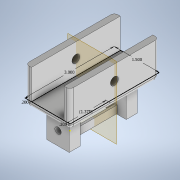
# Autodesk Inventor part: Capillary Holder with O-ring system_rev3_dblOring
Saved by Autodesk Inventor 2020 (Build 240168000, 168)
## iProperties
Created: 2022-02-15
Part Number: Capillary Holder with O-ring system_rev3_dblOring
Material: Generic
Document SubType Name: Modeling
Designer: Beaucage
Density: 1 g/cm^3
Appearance: Default
Author: Beaucage
Autodesk Inventor part; units mm, degrees
ref_plane "YZ Plane" through (0, 0, 0) normal (1, 0, 0) x (0, 1, 0)
ref_plane "XZ Plane" through (0, 0, 0) normal (0, 1, 0) x (-1, 0, 0)
sketch "Sketch1" plane through (0, 0, 0) normal (0, 1, 0) x (-1, 0, 0)
  line L0 (0, 0) -> (38.1, 0)
  line L1 (38.1, 0) -> (38.1, -76.2)
  line L2 (38.1, -76.2) -> (0, -76.2)
  line L3 (0, -76.2) -> (0, 0)
  line L4 (38.1, -76.2) -> (33.02, -76.2)
  line L5 (33.02, -76.2) -> (33.02, 0)
  line L6 (33.02, 0) -> (38.1, 0)
  line L7 (38.1, 0) -> (38.1, -76.2)
  line L8 (0, -76.2) -> (5.08, -76.2)
  line L9 (5.08, -76.2) -> (5.08, 0)
  line L10 (5.08, 0) -> (0, 0)
  line L11 (0, 0) -> (0, -76.2)
  dimension "d0" = 38.1
  dimension "d1" = 76.2
  dimension "d2" = 5.08
  dimension "d3" = 5.08
  constraints: 24 end point, 6 parallel, 3 horizontal, 3 perpendicular, 2 point on line
  measures "d0" distance of L1.end L2.end
  measures "d1" distance of L0.end L1.end
  measures "d2" distance of L5.end L6.end
  measures "d3" distance of L10.end L9.end
extrude "Extrusion1" add sketch "Sketch1" along normal blind 25.4 contours L0 L9 L2 L3 | L0 L1 L2 L5
extrude "Extrusion2" add sketch "Sketch1" against normal blind 5.08
sketch "Sketch2" plane through (0, 25.4, 0) normal (1, 0, 0) x (0, 0, -1)
  line L0 (76.2, 0) -> (0, 0) projected
  line L1 (38.1, 0) -> (38.1, -12.7)
  point P0 (0, -25.4)
  dimension "d8" = 12.7
  constraints: 2 end point, 1 midpoint, 1 vertical
  measures "d8" distance of L1.start L1.end
hole "Hole1" at (0, 12.7, -38.1) direction (-1, 0, 0) diameter 6.7564 end through all clearance for "Socket Head Cap Screw" size "1/4" standard "Ansi Unified Screw Threads"
sketch "Sketch3" plane through (0, -5.08, 0) normal (0, -1, 0) x (1, 0, 0)
  line L0 (0, -76.2) -> (-5.08, -76.2) projected
  line L1 (0, -76.2) -> (0, -63.5)
  line L2 (0, 0) -> (0, -76.2) projected
  line L3 (0, -63.5) -> (0, -38.1)
  line L4 (0, -63.5) -> (-19.05, -63.5)
  line L5 (0, -38.1) -> (-19.05, -38.1)
  line L6 (-38.1, -76.2) -> (-38.1, 0) projected
  line L7 (0, -65.0875) -> (-38.1, -65.0875)
  line L8 (-38.1, -65.0875) -> (-38.1, -61.9125)
  line L9 (-38.1, -61.9125) -> (0, -61.9125)
  line L10 (0, -61.9125) -> (0, -65.0875)
  line L11 (0, -65.0875) -> (-38.1, -61.9125) construction
  line L12 (-38.1, -65.0875) -> (0, -61.9125) construction
  line L13 (0, -36.5125) -> (-38.1, -36.5125)
  line L14 (-38.1, -36.5125) -> (-38.1, -39.6875)
  line L15 (-38.1, -39.6875) -> (0, -39.6875)
  line L16 (0, -39.6875) -> (0, -36.5125)
  line L17 (0, -36.5125) -> (-38.1, -39.6875) construction
  line L18 (-38.1, -36.5125) -> (0, -39.6875) construction
  line L19 (-38.1, 0) -> (-38.1, -76.2) projected
  line L20 (-38.1, 0) -> (0, 0)
  line L21 (0, 0) -> (0, -3.175)
  line L22 (0, -3.175) -> (-38.1, -3.175)
  line L23 (-38.1, -3.175) -> (-38.1, 0)
  line L24 (0, -76.2) -> (-38.1, -76.2)
  line L25 (-38.1, -76.2) -> (-38.1, -73.025)
  line L26 (-38.1, -73.025) -> (0, -73.025)
  line L27 (0, -73.025) -> (0, -76.2)
  line L28 (0, -3.175) -> (0, -15.875)
  line L29 (-38.1, -73.025) -> (-38.1, -60.325)
  line L30 (-38.1, -73.025) -> (-25.4, -73.025) construction
  line L31 (0, -15.875) -> (-38.1, -15.875)
  line L32 (-38.1, -15.875) -> (-38.1, -18.415)
  line L33 (-38.1, -18.415) -> (0, -18.415)
  line L34 (0, -18.415) -> (0, -15.875)
  line L35 (-38.1, -60.325) -> (0.7144, -60.325)
  line L36 (0.7144, -60.325) -> (0.7144, -57.785)
  line L37 (0.7144, -57.785) -> (-38.1, -57.785)
  line L38 (-38.1, -57.785) -> (-38.1, -60.325)
  line L39 (-33.02, 0) -> (-5.08, 0) projected
  line L40 (-38.1, -3.175) -> (-25.4, -3.175)
  line L41 (-25.4, -3.175) -> (-25.4, 0)
  line L42 (-25.4, 0) -> (-38.1, 0)
  line L43 (-38.1, 0) -> (-38.1, -3.175)
  line L44 (0, -3.175) -> (-12.7, -3.175)
  line L45 (-12.7, -3.175) -> (-12.7, 0)
  line L46 (-12.7, 0) -> (0, 0)
  line L47 (0, 0) -> (0, -3.175)
  line L48 (-38.1, -76.2) -> (-25.4, -76.2)
  line L49 (-25.4, -76.2) -> (-25.4, -73.025)
  line L50 (-25.4, -73.025) -> (-38.1, -73.025)
  line L51 (-38.1, -73.025) -> (-38.1, -76.2)
  line L52 (0, -76.2) -> (-12.7, -76.2)
  line L53 (-12.7, -76.2) -> (-12.7, -73.025)
  line L54 (-12.7, -73.025) -> (0, -73.025)
  line L55 (0, -73.025) -> (0, -76.2)
  line L56 (0, -15.875) -> (-9.525, -15.875)
  line L57 (-9.525, -15.875) -> (-9.525, -18.415)
  line L58 (-9.525, -18.415) -> (0, -18.415)
  line L59 (0, -18.415) -> (0, -15.875)
  line L60 (0, -57.785) -> (-9.525, -57.785)
  line L61 (-9.525, -57.785) -> (-9.525, -60.325)
  line L62 (-9.525, -60.325) -> (0, -60.325)
  line L63 (0, -60.325) -> (0, -57.785)
  line L64 (-38.1, -18.415) -> (-28.575, -18.415)
  line L65 (-28.575, -18.415) -> (-28.575, -15.875)
  line L66 (-28.575, -15.875) -> (-38.1, -15.875)
  line L67 (-38.1, -15.875) -> (-38.1, -18.415)
  line L68 (-28.575, -57.785) -> (-38.1, -57.785)
  line L69 (-38.1, -57.785) -> (-38.1, -60.325)
  line L70 (-38.1, -60.325) -> (-28.575, -60.325)
  line L71 (-28.575, -60.325) -> (-28.575, -57.785)
  line L72 (-9.525, -18.415) -> (-28.575, -18.415)
  line L73 (-28.575, -18.415) -> (-28.575, -8.89)
  line L74 (-28.575, -8.89) -> (-9.525, -8.89)
  line L75 (-9.525, -8.89) -> (-9.525, -18.415)
  line L76 (-28.575, -57.785) -> (-9.525, -57.785)
  line L77 (-9.525, -57.785) -> (-9.525, -67.31)
  line L78 (-9.525, -67.31) -> (-28.575, -67.31)
  line L79 (-28.575, -67.31) -> (-28.575, -57.785)
  point P0 (0, -39.6875)
  point P1 (0, -36.5125)
  point P2 (-38.1, -36.5125)
  point P3 (0, -61.9125)
  point P4 (-38.1, -65.0875)
  point P5 (0, -65.0875)
  point P6 (0, -73.025)
  point P7 (-38.1, -18.415)
  point P8 (0, -18.415)
  point P9 (-38.1, -15.875)
  point P10 (0, -57.785)
  point P11 (0, -60.325)
  dimension "d16" = 12.7
  dimension "d17" = 25.4
  dimension "d18" = 19.05
  dimension "d19" = 3.175
  dimension "d20" = 3.175
  dimension "d32" = 3.175
  dimension "d33" = 3.175
  dimension "d34" = 12.7
  dimension "d35" = 12.7
  dimension "d36" = 90
  dimension "d37" = 2.54
  dimension "d38" = 2.54
  dimension "d46" = 12.7
  dimension "d47" = 12.7
  dimension "d48" = 12.7
  dimension "d49" = 9.525
  dimension "d50" = 9.525
  dimension "d51" = 9.525
  constraints: 150 end point, 32 parallel, 19 horizontal, 17 perpendicular, 17 point on line, 5 midpoint, 1 collinear, 3 other
  measures "d16" distance of L0.start L1.end
  measures "d17" distance of L1.end L3.end
  measures "d18" distance of L1.end L4.end
  measures "d19" distance of L7.end L8.end
  measures "d20" distance of L14.end L13.end
  measures "d32" distance of L20.end L21.end
  measures "d33" distance of L24.end L25.end
  measures "d34" distance of L21.end L28.end
  measures "d35" distance of L25.end L29.end
  measures "d36" angle of L30 L29
  measures "d37" distance of L32.end L31.end
  measures "d38" distance of L36.end L35.end
  measures "d46" distance of L42.end L41.end
  measures "d47" distance of L45.end L46.end
  measures "d48" distance of L50.end L30.end
  measures "d49" distance of L66.end L65.end
  measures "d50" distance of L72.end L73.end
  measures "d51" distance of L76.end L77.end
extrude "Extrusion3" add sketch "Sketch3" along normal blind 25.4 contours L77 L78 L79 L7 | L7 L79 L9 L77 | L9 L79 L35 L77 | L35 L71 L37 L61 | L33 L65 L31 L57 | L31 L73 L74 L75
sketch "Sketch4" plane through (-38.1, -5.08, 0) normal (0, 0, 1) x (1, 0, 0)
  line L0 (38.1, -25.4) -> (19.05, -25.4)
  line L1 (19.05, -25.4) -> (19.05, -13.97)
  point P0 (38.1, 5.08)
  dimension "d23" = 11.43
  constraints: 4 end point, 1 vertical
  measures "d23" distance of L0.end L1.end
hole "Hole2" at (-19.05, -19.05, 0) direction (0, 0, -1) diameter 2 end through all
fillet "Fillet1" radius 3.175 8 edges at (-38.1, 10.16, 0) (-19.05, -5.08, 0) (0, 10.16, 0) (-19.05, -5.08, -76.2) (0, 10.16, -76.2) (-38.1, 10.16, -76.2) (0, -5.08, -38.1) (-38.1, -5.08, -38.1)
sketch "Sketch5" plane through (-38.1, -30.48, -57.785) normal (0, 0, 1) x (1, 0, 0)
  line L0 (28.575, 0) -> (9.525, 0) projected
  line L1 (19.05, 0) -> (19.05, 3.175)
  line L2 (19.05, 0.7419) -> (20.955, 0.7419)
  line L3 (20.955, 0.7419) -> (20.955, 7.0919)
  line L4 (20.955, 7.0919) -> (19.05, 7.0919)
  line L5 (19.05, 7.0919) -> (19.05, 0.7419)
  point P0 (38.1, 30.48)
  point P1 (38.8144, 0)
  point P2 (0, 0)
  point P3 (38.1, 0)
  dimension "d39" = 3.175
  dimension "d40" = 1.905
  dimension "d41" = 6.35
  constraints: 10 end point, 2 parallel, 1 horizontal, 1 midpoint, 1 perpendicular, 1 point on line, 1 vertical
  measures "d39" distance of L1.start L1.end
  measures "d40" distance of L4.end L3.end
  measures "d41" distance of L3.end L2.end
extrude "Extrusion4" add sketch "Sketch5" along normal blind 40.64
sketch "Sketch6" plane through (-19.05, -29.7381, -57.785) normal (-1, 0, 0) x (0, 0, 1)
  line L0 (38.4322, 1.5042) -> (1.8474, 1.5042) construction
  line L1 (1.8474, 1.5042) -> (1.8474, 6.5412) construction
  line L2 (1.8474, 6.5412) -> (38.4322, 6.5412) construction
  line L3 (38.4322, 6.5412) -> (38.4322, 1.5042) construction
  spline S0 degree 2 poles (36.9329, 4.7424) (37.2293, 4.7424) (37.7307, 4.5423) (37.9135, 4.3422) knots 0 0 0 1 2 2 2
  spline S1 degree 2 poles (37.9135, 4.3422) (38.0963, 4.1446) (38.2963, 3.5518) (38.2963, 3.1665) knots 0 0 0 1 2 2 2
  spline S2 degree 2 poles (38.2963, 3.1665) (38.2963, 2.7836) (38.1012, 2.2155) (37.916, 2.0056) knots 0 0 0 1 2 2 2
  spline S3 degree 2 poles (37.916, 2.0056) (37.7332, 1.8006) (37.2342, 1.5857) (36.9255, 1.5857) knots 0 0 0 1 2 2 2
  spline S4 degree 2 poles (36.9255, 1.5857) (36.7723, 1.5857) (36.5031, 1.6302) (36.3895, 1.6647) knots 0 0 0 1 2 2 2
  spline S5 degree 2 poles (36.3895, 1.6647) (36.2907, 1.6968) (36.0857, 1.7882) (35.9844, 1.8426) knots 0 0 0 1 2 2 2
  line L4 (35.9844, 1.8426) -> (35.9844, 2.3316)
  line L5 (35.9844, 2.3316) -> (36.0165, 2.3316)
  spline S6 degree 2 poles (36.0165, 2.3316) (36.0709, 2.2822) (36.2388, 2.1439) (36.3598, 2.0772) knots 0 0 0 1 2 2 2
  spline S7 degree 2 poles (36.3598, 2.0772) (36.4759, 2.013) (36.7501, 1.9315) (36.9279, 1.9315) knots 0 0 0 1 2 2 2
  spline S8 degree 2 poles (36.9279, 1.9315) (37.1231, 1.9315) (37.4714, 2.092) (37.6023, 2.2452) knots 0 0 0 1 2 2 2
  spline S9 degree 2 poles (37.6023, 2.2452) (37.7307, 2.4008) (37.874, 2.8726) (37.874, 3.1665) knots 0 0 0 1 2 2 2
  spline S10 degree 2 poles (37.874, 3.1665) (37.874, 3.4802) (37.7233, 3.9322) (37.5924, 4.0878) knots 0 0 0 1 2 2 2
  spline S11 degree 2 poles (37.5924, 4.0878) (37.4639, 4.2385) (37.1206, 4.3916) (36.9279, 4.3916) knots 0 0 0 1 2 2 2
  spline S12 degree 2 poles (36.9279, 4.3916) (36.7526, 4.3916) (36.4537, 4.3052) (36.3376, 4.241) knots 0 0 0 1 2 2 2
  spline S13 degree 2 poles (36.3376, 4.241) (36.2265, 4.1767) (36.061, 4.0434) (36.014, 3.9964) knots 0 0 0 1 2 2 2
  line L6 (36.014, 3.9964) -> (35.9844, 3.9964)
  line L7 (35.9844, 3.9964) -> (35.9844, 4.4805)
  spline S14 degree 2 poles (35.9844, 4.4805) (36.0857, 4.5275) (36.2635, 4.6139) (36.3895, 4.6535) knots 0 0 0 1 2 2 2
  spline S15 degree 2 poles (36.3895, 4.6535) (36.5229, 4.6979) (36.7501, 4.7424) (36.9329, 4.7424) knots 0 0 0 1 2 2 2
  spline S16 degree 2 poles (34.3616, 4.446) (34.4085, 4.4805) (34.5666, 4.6041) (34.6407, 4.6411) knots 0 0 0 1 2 2 2
  spline S17 degree 2 poles (34.6407, 4.6411) (34.742, 4.6954) (34.9322, 4.7523) (35.1051, 4.7523) knots 0 0 0 1 2 2 2
  spline S18 degree 2 poles (35.1051, 4.7523) (35.2459, 4.7523) (35.5003, 4.646) (35.5966, 4.5497) knots 0 0 0 1 2 2 2
  spline S19 degree 2 poles (35.5966, 4.5497) (35.688, 4.4558) (35.7991, 4.1792) (35.7991, 4.0261) knots 0 0 0 1 2 2 2
  spline S20 degree 2 poles (35.7991, 4.0261) (35.7991, 3.7889) (35.5991, 3.453) (35.3817, 3.3567) knots 0 0 0 1 2 2 2
  spline S21 degree 2 poles (35.3817, 3.3567) (35.1891, 3.2678) (34.6654, 3.2011) (34.3616, 3.1838) knots 0 0 0 1 2 2 2
  line L8 (34.3616, 3.1838) -> (34.3616, 3.1097)
  spline S22 degree 2 poles (34.3616, 3.1097) (34.3616, 2.9763) (34.4431, 2.8108) (34.5172, 2.7639) knots 0 0 0 1 2 2 2
  spline S23 degree 2 poles (34.5172, 2.7639) (34.5913, 2.717) (34.8037, 2.6873) (34.9174, 2.6873) knots 0 0 0 1 2 2 2
  spline S24 degree 2 poles (34.9174, 2.6873) (35.0507, 2.6873) (35.4114, 2.7664) (35.5917, 2.8429) knots 0 0 0 1 2 2 2
  line L9 (35.5917, 2.8429) -> (35.6139, 2.8429)
  line L10 (35.6139, 2.8429) -> (35.6139, 2.4502)
  spline S25 degree 2 poles (35.6139, 2.4502) (35.5077, 2.4206) (35.11, 2.3465) (34.9149, 2.3465) knots 0 0 0 1 2 2 2
  spline S26 degree 2 poles (34.9149, 2.3465) (34.6778, 2.3465) (34.3542, 2.4206) (34.2257, 2.5169) knots 0 0 0 1 2 2 2
  spline S27 degree 2 poles (34.2257, 2.5169) (34.0998, 2.6107) (33.9763, 2.9096) (33.9763, 3.1245) knots 0 0 0 1 2 2 2
  line L11 (33.9763, 3.1245) -> (33.9763, 4.688)
  line L12 (33.9763, 4.688) -> (34.3616, 4.688)
  line L13 (34.3616, 4.688) -> (34.3616, 4.446)
  line L14 (34.3616, 4.1249) -> (34.3616, 3.4901)
  spline S28 degree 2 poles (34.3616, 3.4901) (34.4999, 3.5024) (34.9174, 3.5444) (35.0483, 3.5839) knots 0 0 0 1 2 2 2
  spline S29 degree 2 poles (35.0483, 3.5839) (35.2014, 3.6309) (35.4015, 3.826) (35.4015, 3.9989) knots 0 0 0 1 2 2 2
  spline S30 degree 2 poles (35.4015, 3.9989) (35.4015, 4.1965) (35.1792, 4.3966) (34.9668, 4.3966) knots 0 0 0 1 2 2 2
  spline S31 degree 2 poles (34.9668, 4.3966) (34.7864, 4.3966) (34.49, 4.241) (34.3616, 4.1249) knots 0 0 0 1 2 2 2
  line L15 (33.0426, 4.688) -> (33.4279, 4.688)
  line L16 (33.4279, 4.688) -> (33.4279, 1.5042)
  line L17 (33.4279, 1.5042) -> (33.0426, 1.5042)
  line L18 (33.0426, 1.5042) -> (33.0426, 4.688)
  line L19 (32.0842, 4.688) -> (32.4696, 4.688)
  line L20 (32.4696, 4.688) -> (32.4696, 2.4008)
  line L21 (32.4696, 2.4008) -> (32.0842, 2.4008)
  line L22 (32.0842, 2.4008) -> (32.0842, 4.688)
  line L23 (32.0571, 2.0204) -> (32.4943, 2.0204)
  line L24 (32.4943, 2.0204) -> (32.4943, 1.6203)
  line L25 (32.4943, 1.6203) -> (32.0571, 1.6203)
  line L26 (32.0571, 1.6203) -> (32.0571, 2.0204)
  spline S32 degree 2 poles (29.6019, 3.5074) (29.6019, 4.0681) (30.1453, 4.7523) (30.5553, 4.7523) knots 0 0 0 1 2 2 2
  spline S33 degree 2 poles (30.5553, 4.7523) (30.7406, 4.7523) (31.0048, 4.6609) (31.1333, 4.5818) knots 0 0 0 1 2 2 2
  line L27 (31.1333, 4.5818) -> (31.158, 4.688)
  line L28 (31.158, 4.688) -> (31.5186, 4.688)
  line L29 (31.5186, 4.688) -> (31.5186, 1.5042)
  line L30 (31.5186, 1.5042) -> (31.1333, 1.5042)
  line L31 (31.1333, 1.5042) -> (31.1333, 2.6404)
  spline S34 degree 2 poles (31.1333, 2.6404) (30.9876, 2.5095) (30.6492, 2.3366) (30.4343, 2.3366) knots 0 0 0 1 2 2 2
  spline S35 degree 2 poles (30.4343, 2.3366) (30.0465, 2.3366) (29.6019, 2.9565) (29.6019, 3.5074) knots 0 0 0 1 2 2 2
  spline S36 degree 2 poles (29.9996, 3.537) (29.9996, 3.127) (30.249, 2.7021) (30.5257, 2.7021) knots 0 0 0 1 2 2 2
  spline S37 degree 2 poles (30.5257, 2.7021) (30.6813, 2.7021) (31.0024, 2.8503) (31.1333, 2.964) knots 0 0 0 1 2 2 2
  line L32 (31.1333, 2.964) -> (31.1333, 4.2755)
  spline S38 degree 2 poles (31.1333, 4.2755) (30.9876, 4.3472) (30.7628, 4.4064) (30.6294, 4.4064) knots 0 0 0 1 2 2 2
  spline S39 degree 2 poles (30.6294, 4.4064) (30.3355, 4.4064) (29.9996, 3.989) (29.9996, 3.537) knots 0 0 0 1 2 2 2
  line L33 (27.989, 2.8133) -> (28.0087, 2.8133)
  spline S40 degree 2 poles (28.0087, 2.8133) (28.0532, 2.8009) (28.1495, 2.796) (28.2162, 2.796) knots 0 0 0 1 2 2 2
  spline S41 degree 2 poles (28.2162, 2.796) (28.3718, 2.796) (28.6781, 2.9318) (28.8164, 3.0652) knots 0 0 0 1 2 2 2
  line L34 (28.8164, 3.0652) -> (28.8164, 4.688)
  line L35 (28.8164, 4.688) -> (29.2017, 4.688)
  line L36 (29.2017, 4.688) -> (29.2017, 2.4008)
  line L37 (29.2017, 2.4008) -> (28.8164, 2.4008)
  line L38 (28.8164, 2.4008) -> (28.8164, 2.7417)
  spline S42 degree 2 poles (28.8164, 2.7417) (28.6065, 2.5539) (28.2928, 2.4008) (28.1446, 2.4008) knots 0 0 0 1 2 2 2
  spline S43 degree 2 poles (28.1446, 2.4008) (28.0853, 2.4008) (28.026, 2.4057) (27.989, 2.4131) knots 0 0 0 1 2 2 2
  line L39 (27.989, 2.4131) -> (27.989, 2.8133)
  spline S44 degree 2 poles (26.4156, 4.446) (26.4625, 4.4805) (26.6206, 4.6041) (26.6947, 4.6411) knots 0 0 0 1 2 2 2
  spline S45 degree 2 poles (26.6947, 4.6411) (26.7959, 4.6954) (26.9861, 4.7523) (27.159, 4.7523) knots 0 0 0 1 2 2 2
  spline S46 degree 2 poles (27.159, 4.7523) (27.2998, 4.7523) (27.5542, 4.646) (27.6506, 4.5497) knots 0 0 0 1 2 2 2
  spline S47 degree 2 poles (27.6506, 4.5497) (27.742, 4.4558) (27.8531, 4.1792) (27.8531, 4.0261) knots 0 0 0 1 2 2 2
  spline S48 degree 2 poles (27.8531, 4.0261) (27.8531, 3.7889) (27.653, 3.453) (27.4357, 3.3567) knots 0 0 0 1 2 2 2
  spline S49 degree 2 poles (27.4357, 3.3567) (27.243, 3.2678) (26.7194, 3.2011) (26.4156, 3.1838) knots 0 0 0 1 2 2 2
  line L40 (26.4156, 3.1838) -> (26.4156, 3.1097)
  spline S50 degree 2 poles (26.4156, 3.1097) (26.4156, 2.9763) (26.4971, 2.8108) (26.5712, 2.7639) knots 0 0 0 1 2 2 2
  spline S51 degree 2 poles (26.5712, 2.7639) (26.6453, 2.717) (26.8577, 2.6873) (26.9713, 2.6873) knots 0 0 0 1 2 2 2
  spline S52 degree 2 poles (26.9713, 2.6873) (27.1047, 2.6873) (27.4653, 2.7664) (27.6456, 2.8429) knots 0 0 0 1 2 2 2
  line L41 (27.6456, 2.8429) -> (27.6679, 2.8429)
  line L42 (27.6679, 2.8429) -> (27.6679, 2.4502)
  spline S53 degree 2 poles (27.6679, 2.4502) (27.5616, 2.4206) (27.164, 2.3465) (26.9688, 2.3465) knots 0 0 0 1 2 2 2
  spline S54 degree 2 poles (26.9688, 2.3465) (26.7317, 2.3465) (26.4081, 2.4206) (26.2797, 2.5169) knots 0 0 0 1 2 2 2
  spline S55 degree 2 poles (26.2797, 2.5169) (26.1537, 2.6107) (26.0302, 2.9096) (26.0302, 3.1245) knots 0 0 0 1 2 2 2
  line L43 (26.0302, 3.1245) -> (26.0302, 4.688)
  line L44 (26.0302, 4.688) -> (26.4156, 4.688)
  line L45 (26.4156, 4.688) -> (26.4156, 4.446)
  line L46 (26.4156, 4.1249) -> (26.4156, 3.4901)
  spline S56 degree 2 poles (26.4156, 3.4901) (26.5539, 3.5024) (26.9713, 3.5444) (27.1022, 3.5839) knots 0 0 0 1 2 2 2
  spline S57 degree 2 poles (27.1022, 3.5839) (27.2554, 3.6309) (27.4554, 3.826) (27.4554, 3.9989) knots 0 0 0 1 2 2 2
  spline S58 degree 2 poles (27.4554, 3.9989) (27.4554, 4.1965) (27.2331, 4.3966) (27.0207, 4.3966) knots 0 0 0 1 2 2 2
  spline S59 degree 2 poles (27.0207, 4.3966) (26.8404, 4.3966) (26.544, 4.241) (26.4156, 4.1249) knots 0 0 0 1 2 2 2
  line L47 (23.6936, 4.688) -> (24.0789, 4.688)
  line L48 (24.0789, 4.688) -> (24.0789, 3.3839)
  spline S60 degree 2 poles (24.0789, 3.3839) (24.0789, 3.2258) (24.1086, 2.9541) (24.153, 2.8726) knots 0 0 0 1 2 2 2
  spline S61 degree 2 poles (24.153, 2.8726) (24.2, 2.7861) (24.3679, 2.7021) (24.5112, 2.7021) knots 0 0 0 1 2 2 2
  spline S62 degree 2 poles (24.5112, 2.7021) (24.6544, 2.7021) (24.9582, 2.8553) (25.104, 2.9788) knots 0 0 0 1 2 2 2
  line L49 (25.104, 2.9788) -> (25.104, 4.688)
  line L50 (25.104, 4.688) -> (25.4893, 4.688)
  line L51 (25.4893, 4.688) -> (25.4893, 2.4008)
  line L52 (25.4893, 2.4008) -> (25.104, 2.4008)
  line L53 (25.104, 2.4008) -> (25.104, 2.6552)
  spline S63 degree 2 poles (25.104, 2.6552) (24.9311, 2.4996) (24.5976, 2.3366) (24.4099, 2.3366) knots 0 0 0 1 2 2 2
  spline S64 degree 2 poles (24.4099, 2.3366) (24.074, 2.3366) (23.6936, 2.7812) (23.6936, 3.2036) knots 0 0 0 1 2 2 2
  line L54 (23.6936, 3.2036) -> (23.6936, 4.688)
  spline S65 degree 2 poles (22.4611, 4.7325) (22.7748, 4.7325) (23.128, 4.3743) (23.128, 3.9865) knots 0 0 0 1 2 2 2
  line L55 (23.128, 3.9865) -> (23.128, 2.7194)
  line L56 (23.128, 2.7194) -> (23.3873, 2.7194)
  line L57 (23.3873, 2.7194) -> (23.3873, 2.4008)
  line L58 (23.3873, 2.4008) -> (23.128, 2.4008)
  line L59 (23.128, 2.4008) -> (23.128, 1.7438)
  line L60 (23.128, 1.7438) -> (22.7426, 1.7438)
  line L61 (22.7426, 1.7438) -> (22.7426, 2.4008)
  line L62 (22.7426, 2.4008) -> (22.0337, 2.4008)
  line L63 (22.0337, 2.4008) -> (22.0337, 2.7194)
  line L64 (22.0337, 2.7194) -> (22.7426, 2.7194)
  line L65 (22.7426, 2.7194) -> (22.7426, 3.8087)
  spline S66 degree 2 poles (22.7426, 3.8087) (22.7426, 3.9816) (22.7303, 4.1718) (22.6883, 4.2533) knots 0 0 0 1 2 2 2
  spline S67 degree 2 poles (22.6883, 4.2533) (22.6537, 4.3249) (22.4981, 4.3966) (22.3647, 4.3966) knots 0 0 0 1 2 2 2
  spline S68 degree 2 poles (22.3647, 4.3966) (22.2709, 4.3966) (22.0955, 4.3398) (22.056, 4.3225) knots 0 0 0 1 2 2 2
  line L66 (22.056, 4.3225) -> (22.0337, 4.3225)
  line L67 (22.0337, 4.3225) -> (22.0337, 4.6683)
  spline S69 degree 2 poles (22.0337, 4.6683) (22.1424, 4.6979) (22.3647, 4.7325) (22.4611, 4.7325) knots 0 0 0 1 2 2 2
  spline S70 degree 2 poles (21.1322, 4.7424) (21.3619, 4.7424) (21.7596, 4.6189) (21.8905, 4.5497) knots 0 0 0 1 2 2 2
  line L68 (21.8905, 4.5497) -> (21.8905, 4.1175)
  line L69 (21.8905, 4.1175) -> (21.8707, 4.1175)
  spline S71 degree 2 poles (21.8707, 4.1175) (21.8213, 4.157) (21.6879, 4.2508) (21.5768, 4.3027) knots 0 0 0 1 2 2 2
  spline S72 degree 2 poles (21.5768, 4.3027) (21.4805, 4.3496) (21.2433, 4.4188) (21.1174, 4.4188) knots 0 0 0 1 2 2 2
  spline S73 degree 2 poles (21.1174, 4.4188) (21.026, 4.4188) (20.816, 4.3768) (20.7666, 4.3422) knots 0 0 0 1 2 2 2
  spline S74 degree 2 poles (20.7666, 4.3422) (20.695, 4.2953) (20.6308, 4.1891) (20.6308, 4.0804) knots 0 0 0 1 2 2 2
  spline S75 degree 2 poles (20.6308, 4.0804) (20.6308, 3.9446) (20.779, 3.8038) (20.9692, 3.7568) knots 0 0 0 1 2 2 2
  spline S76 degree 2 poles (20.9692, 3.7568) (21.0433, 3.7395) (21.2804, 3.6901) (21.3817, 3.663) knots 0 0 0 1 2 2 2
  spline S77 degree 2 poles (21.3817, 3.663) (21.6435, 3.5864) (21.8806, 3.2702) (21.8806, 3.0455) knots 0 0 0 1 2 2 2
  spline S78 degree 2 poles (21.8806, 3.0455) (21.8806, 2.7342) (21.4138, 2.3465) (21.0285, 2.3465) knots 0 0 0 1 2 2 2
  spline S79 degree 2 poles (21.0285, 2.3465) (20.8383, 2.3465) (20.4529, 2.4403) (20.322, 2.5119) knots 0 0 0 1 2 2 2
  line L70 (20.322, 2.5119) -> (20.322, 2.9244)
  line L71 (20.322, 2.9244) -> (20.3418, 2.9244)
  spline S80 degree 2 poles (20.3418, 2.9244) (20.49, 2.8059) (20.8506, 2.67) (21.0359, 2.67) knots 0 0 0 1 2 2 2
  spline S81 degree 2 poles (21.0359, 2.67) (21.2261, 2.67) (21.4879, 2.8306) (21.4879, 2.9911) knots 0 0 0 1 2 2 2
  spline S82 degree 2 poles (21.4879, 2.9911) (21.4879, 3.1369) (21.3323, 3.2777) (21.1594, 3.3221) knots 0 0 0 1 2 2 2
  spline S83 degree 2 poles (21.1594, 3.3221) (21.0754, 3.3443) (20.863, 3.3888) (20.7469, 3.416) knots 0 0 0 1 2 2 2
  spline S84 degree 2 poles (20.7469, 3.416) (20.4949, 3.4802) (20.238, 3.7741) (20.238, 4.0285) knots 0 0 0 1 2 2 2
  spline S85 degree 2 poles (20.238, 4.0285) (20.238, 4.1767) (20.3541, 4.4386) (20.4678, 4.5349) knots 0 0 0 1 2 2 2
  spline S86 degree 2 poles (20.4678, 4.5349) (20.5888, 4.6362) (20.8975, 4.7424) (21.1322, 4.7424) knots 0 0 0 1 2 2 2
  spline S87 degree 2 poles (17.8792, 4.7325) (18.1929, 4.7325) (18.5461, 4.3743) (18.5461, 3.9865) knots 0 0 0 1 2 2 2
  line L72 (18.5461, 3.9865) -> (18.5461, 2.7194)
  line L73 (18.5461, 2.7194) -> (18.8054, 2.7194)
  line L74 (18.8054, 2.7194) -> (18.8054, 2.4008)
  line L75 (18.8054, 2.4008) -> (18.5461, 2.4008)
  line L76 (18.5461, 2.4008) -> (18.5461, 1.7438)
  line L77 (18.5461, 1.7438) -> (18.1608, 1.7438)
  line L78 (18.1608, 1.7438) -> (18.1608, 2.4008)
  line L79 (18.1608, 2.4008) -> (17.4519, 2.4008)
  line L80 (17.4519, 2.4008) -> (17.4519, 2.7194)
  line L81 (17.4519, 2.7194) -> (18.1608, 2.7194)
  line L82 (18.1608, 2.7194) -> (18.1608, 3.8087)
  spline S88 degree 2 poles (18.1608, 3.8087) (18.1608, 3.9816) (18.1484, 4.1718) (18.1064, 4.2533) knots 0 0 0 1 2 2 2
  spline S89 degree 2 poles (18.1064, 4.2533) (18.0718, 4.3249) (17.9162, 4.3966) (17.7829, 4.3966) knots 0 0 0 1 2 2 2
  spline S90 degree 2 poles (17.7829, 4.3966) (17.689, 4.3966) (17.5136, 4.3398) (17.4741, 4.3225) knots 0 0 0 1 2 2 2
  line L83 (17.4741, 4.3225) -> (17.4519, 4.3225)
  line L84 (17.4519, 4.3225) -> (17.4519, 4.6683)
  spline S91 degree 2 poles (17.4519, 4.6683) (17.5605, 4.6979) (17.7829, 4.7325) (17.8792, 4.7325) knots 0 0 0 1 2 2 2
  line L85 (15.3721, 4.688) -> (15.7574, 4.688)
  line L86 (15.7574, 4.688) -> (15.7574, 3.3839)
  spline S92 degree 2 poles (15.7574, 3.3839) (15.7574, 3.2258) (15.7871, 2.9541) (15.8315, 2.8726) knots 0 0 0 1 2 2 2
  spline S93 degree 2 poles (15.8315, 2.8726) (15.8785, 2.7861) (16.0464, 2.7021) (16.1897, 2.7021) knots 0 0 0 1 2 2 2
  spline S94 degree 2 poles (16.1897, 2.7021) (16.333, 2.7021) (16.6368, 2.8553) (16.7825, 2.9788) knots 0 0 0 1 2 2 2
  line L87 (16.7825, 2.9788) -> (16.7825, 4.688)
  line L88 (16.7825, 4.688) -> (17.1678, 4.688)
  line L89 (17.1678, 4.688) -> (17.1678, 1.5042)
  line L90 (17.1678, 1.5042) -> (16.7825, 1.5042)
  line L91 (16.7825, 1.5042) -> (16.7825, 2.6552)
  spline S95 degree 2 poles (16.7825, 2.6552) (16.6096, 2.4996) (16.2761, 2.3366) (16.0884, 2.3366) knots 0 0 0 1 2 2 2
  spline S96 degree 2 poles (16.0884, 2.3366) (15.7525, 2.3366) (15.3721, 2.7812) (15.3721, 3.2036) knots 0 0 0 1 2 2 2
  line L92 (15.3721, 3.2036) -> (15.3721, 4.688)
  line L93 (14.4384, 4.688) -> (14.8238, 4.688)
  line L94 (14.8238, 4.688) -> (14.8238, 2.4008)
  line L95 (14.8238, 2.4008) -> (14.4384, 2.4008)
  line L96 (14.4384, 2.4008) -> (14.4384, 4.688)
  line L97 (14.4113, 2.0204) -> (14.8485, 2.0204)
  line L98 (14.8485, 2.0204) -> (14.8485, 1.6203)
  line L99 (14.8485, 1.6203) -> (14.4113, 1.6203)
  line L100 (14.4113, 1.6203) -> (14.4113, 2.0204)
  spline S97 degree 2 poles (13.2553, 4.7424) (13.485, 4.7424) (13.8827, 4.6189) (14.0136, 4.5497) knots 0 0 0 1 2 2 2
  line L101 (14.0136, 4.5497) -> (14.0136, 4.1175)
  line L102 (14.0136, 4.1175) -> (13.9938, 4.1175)
  spline S98 degree 2 poles (13.9938, 4.1175) (13.9444, 4.157) (13.8111, 4.2508) (13.6999, 4.3027) knots 0 0 0 1 2 2 2
  spline S99 degree 2 poles (13.6999, 4.3027) (13.6036, 4.3496) (13.3665, 4.4188) (13.2405, 4.4188) knots 0 0 0 1 2 2 2
  spline S100 degree 2 poles (13.2405, 4.4188) (13.1491, 4.4188) (12.9391, 4.3768) (12.8897, 4.3422) knots 0 0 0 1 2 2 2
  spline S101 degree 2 poles (12.8897, 4.3422) (12.8181, 4.2953) (12.7539, 4.1891) (12.7539, 4.0804) knots 0 0 0 1 2 2 2
  spline S102 degree 2 poles (12.7539, 4.0804) (12.7539, 3.9446) (12.9021, 3.8038) (13.0923, 3.7568) knots 0 0 0 1 2 2 2
  spline S103 degree 2 poles (13.0923, 3.7568) (13.1664, 3.7395) (13.4035, 3.6901) (13.5048, 3.663) knots 0 0 0 1 2 2 2
  spline S104 degree 2 poles (13.5048, 3.663) (13.7666, 3.5864) (14.0037, 3.2702) (14.0037, 3.0455) knots 0 0 0 1 2 2 2
  spline S105 degree 2 poles (14.0037, 3.0455) (14.0037, 2.7342) (13.5369, 2.3465) (13.1516, 2.3465) knots 0 0 0 1 2 2 2
  spline S106 degree 2 poles (13.1516, 2.3465) (12.9614, 2.3465) (12.5761, 2.4403) (12.4451, 2.5119) knots 0 0 0 1 2 2 2
  line L103 (12.4451, 2.5119) -> (12.4451, 2.9244)
  line L104 (12.4451, 2.9244) -> (12.4649, 2.9244)
  spline S107 degree 2 poles (12.4649, 2.9244) (12.6131, 2.8059) (12.9737, 2.67) (13.159, 2.67) knots 0 0 0 1 2 2 2
  spline S108 degree 2 poles (13.159, 2.67) (13.3492, 2.67) (13.611, 2.8306) (13.611, 2.9911) knots 0 0 0 1 2 2 2
  spline S109 degree 2 poles (13.611, 2.9911) (13.611, 3.1369) (13.4554, 3.2777) (13.2825, 3.3221) knots 0 0 0 1 2 2 2
  spline S110 degree 2 poles (13.2825, 3.3221) (13.1985, 3.3443) (12.9861, 3.3888) (12.87, 3.416) knots 0 0 0 1 2 2 2
  spline S111 degree 2 poles (12.87, 3.416) (12.618, 3.4802) (12.3612, 3.7741) (12.3612, 4.0285) knots 0 0 0 1 2 2 2
  spline S112 degree 2 poles (12.3612, 4.0285) (12.3612, 4.1767) (12.4773, 4.4386) (12.5909, 4.5349) knots 0 0 0 1 2 2 2
  spline S113 degree 2 poles (12.5909, 4.5349) (12.7119, 4.6362) (13.0207, 4.7424) (13.2553, 4.7424) knots 0 0 0 1 2 2 2
  spline S114 degree 2 poles (10.0764, 4.7424) (10.3061, 4.7424) (10.7038, 4.6189) (10.8347, 4.5497) knots 0 0 0 1 2 2 2
  line L105 (10.8347, 4.5497) -> (10.8347, 4.1175)
  line L106 (10.8347, 4.1175) -> (10.8149, 4.1175)
  spline S115 degree 2 poles (10.8149, 4.1175) (10.7655, 4.157) (10.6322, 4.2508) (10.521, 4.3027) knots 0 0 0 1 2 2 2
  spline S116 degree 2 poles (10.521, 4.3027) (10.4247, 4.3496) (10.1876, 4.4188) (10.0616, 4.4188) knots 0 0 0 1 2 2 2
  spline S117 degree 2 poles (10.0616, 4.4188) (9.9702, 4.4188) (9.7602, 4.3768) (9.7108, 4.3422) knots 0 0 0 1 2 2 2
  spline S118 degree 2 poles (9.7108, 4.3422) (9.6392, 4.2953) (9.575, 4.1891) (9.575, 4.0804) knots 0 0 0 1 2 2 2
  spline S119 degree 2 poles (9.575, 4.0804) (9.575, 3.9446) (9.7232, 3.8038) (9.9134, 3.7568) knots 0 0 0 1 2 2 2
  spline S120 degree 2 poles (9.9134, 3.7568) (9.9875, 3.7395) (10.2246, 3.6901) (10.3259, 3.663) knots 0 0 0 1 2 2 2
  spline S121 degree 2 poles (10.3259, 3.663) (10.5877, 3.5864) (10.8248, 3.2702) (10.8248, 3.0455) knots 0 0 0 1 2 2 2
  spline S122 degree 2 poles (10.8248, 3.0455) (10.8248, 2.7342) (10.358, 2.3465) (9.9727, 2.3465) knots 0 0 0 1 2 2 2
  spline S123 degree 2 poles (9.9727, 2.3465) (9.7825, 2.3465) (9.3971, 2.4403) (9.2662, 2.5119) knots 0 0 0 1 2 2 2
  line L107 (9.2662, 2.5119) -> (9.2662, 2.9244)
  line L108 (9.2662, 2.9244) -> (9.286, 2.9244)
  spline S124 degree 2 poles (9.286, 2.9244) (9.4342, 2.8059) (9.7948, 2.67) (9.9801, 2.67) knots 0 0 0 1 2 2 2
  spline S125 degree 2 poles (9.9801, 2.67) (10.1703, 2.67) (10.4321, 2.8306) (10.4321, 2.9911) knots 0 0 0 1 2 2 2
  spline S126 degree 2 poles (10.4321, 2.9911) (10.4321, 3.1369) (10.2765, 3.2777) (10.1036, 3.3221) knots 0 0 0 1 2 2 2
  spline S127 degree 2 poles (10.1036, 3.3221) (10.0196, 3.3443) (9.8072, 3.3888) (9.6911, 3.416) knots 0 0 0 1 2 2 2
  spline S128 degree 2 poles (9.6911, 3.416) (9.4391, 3.4802) (9.1823, 3.7741) (9.1823, 4.0285) knots 0 0 0 1 2 2 2
  spline S129 degree 2 poles (9.1823, 4.0285) (9.1823, 4.1767) (9.2983, 4.4386) (9.412, 4.5349) knots 0 0 0 1 2 2 2
  spline S130 degree 2 poles (9.412, 4.5349) (9.533, 4.6362) (9.8417, 4.7424) (10.0764, 4.7424) knots 0 0 0 1 2 2 2
  line L109 (8.4314, 4.688) -> (8.8167, 4.688)
  line L110 (8.8167, 4.688) -> (8.8167, 2.4008)
  line L111 (8.8167, 2.4008) -> (8.4314, 2.4008)
  line L112 (8.4314, 2.4008) -> (8.4314, 4.688)
  line L113 (8.4042, 2.0204) -> (8.8414, 2.0204)
  line L114 (8.8414, 2.0204) -> (8.8414, 1.6203)
  line L115 (8.8414, 1.6203) -> (8.4042, 1.6203)
  line L116 (8.4042, 1.6203) -> (8.4042, 2.0204)
  line L117 (6.1071, 4.688) -> (6.4924, 4.688)
  line L118 (6.4924, 4.688) -> (6.4924, 4.4558)
  spline S131 degree 2 poles (6.4924, 4.4558) (6.5813, 4.5299) (6.7122, 4.6288) (6.8012, 4.6707) knots 0 0 0 1 2 2 2
  spline S132 degree 2 poles (6.8012, 4.6707) (6.8827, 4.7103) (7.058, 4.7523) (7.1741, 4.7523) knots 0 0 0 1 2 2 2
  spline S133 degree 2 poles (7.1741, 4.7523) (7.3619, 4.7523) (7.678, 4.5966) (7.7892, 4.446) knots 0 0 0 1 2 2 2
  spline S134 degree 2 poles (7.7892, 4.446) (7.9003, 4.2953) (8.0238, 3.8507) (8.0238, 3.5617) knots 0 0 0 1 2 2 2
  spline S135 degree 2 poles (8.0238, 3.5617) (8.0238, 3.2604) (7.8682, 2.8207) (7.7324, 2.6552) knots 0 0 0 1 2 2 2
  spline S136 degree 2 poles (7.7324, 2.6552) (7.6064, 2.507) (7.2532, 2.3366) (7.058, 2.3366) knots 0 0 0 1 2 2 2
  spline S137 degree 2 poles (7.058, 2.3366) (6.8876, 2.3366) (6.6332, 2.4131) (6.4924, 2.4922) knots 0 0 0 1 2 2 2
  line L119 (6.4924, 2.4922) -> (6.4924, 1.5042)
  line L120 (6.4924, 1.5042) -> (6.1071, 1.5042)
  line L121 (6.1071, 1.5042) -> (6.1071, 4.688)
  line L122 (6.4924, 4.1323) -> (6.4924, 2.8108)
  spline S138 degree 2 poles (6.4924, 2.8108) (6.6357, 2.7417) (6.8629, 2.6898) (6.9938, 2.6898) knots 0 0 0 1 2 2 2
  spline S139 degree 2 poles (6.9938, 2.6898) (7.2902, 2.6898) (7.6261, 3.1344) (7.6261, 3.5543) knots 0 0 0 1 2 2 2
  spline S140 degree 2 poles (7.6261, 3.5543) (7.6261, 3.9594) (7.3693, 4.3867) (7.0852, 4.3867) knots 0 0 0 1 2 2 2
  spline S141 degree 2 poles (7.0852, 4.3867) (6.9345, 4.3867) (6.6283, 4.2484) (6.4924, 4.1323) knots 0 0 0 1 2 2 2
  spline S142 degree 2 poles (4.5559, 4.7399) (5.1043, 4.7399) (5.7069, 4.1249) (5.7069, 3.5568) knots 0 0 0 1 2 2 2
  spline S143 degree 2 poles (5.7069, 3.5568) (5.7069, 2.9985) (5.1215, 2.3366) (4.6498, 2.3366) knots 0 0 0 1 2 2 2
  spline S144 degree 2 poles (4.6498, 2.3366) (4.4374, 2.3366) (4.1088, 2.4601) (3.9878, 2.591) knots 0 0 0 1 2 2 2
  spline S145 degree 2 poles (3.9878, 2.591) (3.8643, 2.7219) (3.7334, 3.0998) (3.7334, 3.374) knots 0 0 0 1 2 2 2
  line L123 (3.7334, 3.374) -> (3.7334, 3.5839)
  line L124 (3.7334, 3.5839) -> (5.3167, 3.5839)
  spline S146 degree 2 poles (5.3167, 3.5839) (5.3167, 3.9816) (4.9165, 4.404) (4.5609, 4.404) knots 0 0 0 1 2 2 2
  spline S147 degree 2 poles (4.5609, 4.404) (4.4349, 4.404) (4.1904, 4.3472) (4.0916, 4.3027) knots 0 0 0 1 2 2 2
  spline S148 degree 2 poles (4.0916, 4.3027) (3.9878, 4.2533) (3.8445, 4.1669) (3.7976, 4.1273) knots 0 0 0 1 2 2 2
  line L125 (3.7976, 4.1273) -> (3.7754, 4.1273)
  line L126 (3.7754, 4.1273) -> (3.7754, 4.5472)
  spline S149 degree 2 poles (3.7754, 4.5472) (3.8421, 4.5744) (4.0446, 4.6535) (4.1237, 4.6757) knots 0 0 0 1 2 2 2
  spline S150 degree 2 poles (4.1237, 4.6757) (4.2348, 4.7078) (4.4176, 4.7399) (4.5559, 4.7399) knots 0 0 0 1 2 2 2
  spline S151 degree 2 poles (4.1088, 3.29) (4.1138, 3.1344) (4.178, 2.9071) (4.2398, 2.8306) knots 0 0 0 1 2 2 2
  spline S152 degree 2 poles (4.2398, 2.8306) (4.3064, 2.7441) (4.5164, 2.6527) (4.672, 2.6527) knots 0 0 0 1 2 2 2
  spline S153 degree 2 poles (4.672, 2.6527) (4.8251, 2.6527) (5.04, 2.7441) (5.129, 2.833) knots 0 0 0 1 2 2 2
  spline S154 degree 2 poles (5.129, 2.833) (5.2154, 2.9244) (5.3043, 3.1443) (5.3167, 3.29) knots 0 0 0 1 2 2 2
  line L127 (5.3167, 3.29) -> (4.1088, 3.29)
  line L128 (2.6985, 1.64) -> (2.7553, 3.8482)
  line L129 (2.7553, 3.8482) -> (3.0937, 3.8482)
  line L130 (3.0937, 3.8482) -> (3.1554, 1.64)
  line L131 (3.1554, 1.64) -> (2.6985, 1.64)
  line L132 (2.7182, 4.688) -> (3.1357, 4.688)
  line L133 (3.1357, 4.688) -> (3.1357, 4.2558)
  line L134 (3.1357, 4.2558) -> (2.7182, 4.2558)
  line L135 (2.7182, 4.2558) -> (2.7182, 4.688)
  point P0 (57.785, 29.7381)
  constraints: 2 other
extrude "Extrusion5" cut sketch "Sketch6" against normal blind 1.27
sketch "Sketch7" plane through (-28.575, -5.08, -8.89) normal (0, 0, 1) x (1, 0, 0)
  circle A0 centre (9.525, -13.97) radius 1 projected
  point P0 (28.575, 5.08)
hole "Hole3" at (-19.05, -19.05, -8.89) direction (0, 0, -1) diameter 5.4102 depth 6.35
sketch "Sketch8" plane through (-19.05, -19.05, -15.24) normal (0, 0, 1) x (1, 0, 0)
  circle A0 centre (0, 0) radius 1 projected
  point P0 (19.05, 19.05)
hole "Hole4" at (-19.05, -19.05, -15.24) direction (0, 0, -1) diameter 4.4704 depth 2.032
sketch "Sketch9" plane through (0, -5.08, 0) normal (0, -1, 0) x (1, 0, 0)
  line L0 (-3.175, -3.175) -> (-3.175, -73.025) projected
  line L1 (-3.175, -3.175) -> (-3.175, -38.1)
  point P0 (0, 0)
  dimension "d66" = 34.925
  constraints: 2 end point, 1 midpoint
  measures "d66" distance of L0.start L1.end
ref_plane "Work Plane1" through (-3.175, -5.08, -38.1) normal (0, 0, 1) x (1, 0, 0)
mirror "Mirror1" about plane through (-3.175, -5.08, -38.1) normal (0, 0, 1) of "Hole3", "Hole4"
body "Solid1"
